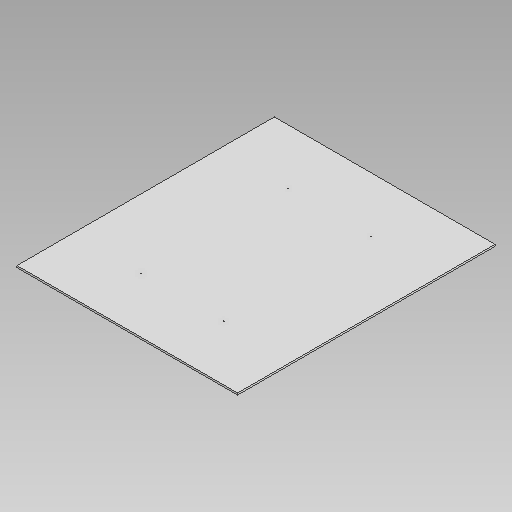
# Autodesk Inventor part: cover_base
Saved by Autodesk Inventor 2021 (Build 250183000, 183)
## iProperties
Created: 2021-05-06
Part Number: cover_base
Material: Generic
Document SubType Name: Modeling
Designer: Watchdog
Density: 1 g/cm^3
Appearance: Default
Author: Watchdog
Autodesk Inventor part; units mm, degrees
ref_plane "YZ Plane" through (0, 0, 0) normal (1, 0, 0) x (0, 1, 0)
ref_plane "XZ Plane" through (0, 0, 0) normal (0, 1, 0) x (-1, 0, 0)
ref_plane "XY Plane" through (0, 0, 0) normal (0, 0, 1) x (1, 0, 0)
sketch "Sketch1" plane through (0, 0, 0) normal (0, 1, 0) x (-1, 0, 0)
  line L0 (600, 700) -> (-600, 700)
  line L1 (-600, 700) -> (-600, -700)
  line L2 (-600, -700) -> (600, -700)
  line L3 (600, -700) -> (600, 700)
  point P0 (0, 0)
  dimension "d0" = 700
  dimension "d1" = 1400
  dimension "d2" = 1200
  dimension "d3" = 600
  constraints: 8 end point, 2 parallel, 1 horizontal, 1 perpendicular
  measures "d0" distance from line of point (0, 0) L0
  measures "d1" distance between parallel lines of L2 L0
  measures "d2" distance between parallel lines of L1 L3
  measures "d3" distance from line of point (0, 0) L3
extrude "base" add sketch "Sketch1" along normal blind 10
sketch "Sketch2" plane through (0, 10, 0) normal (0, 1, 0) x (1, 0, 0)
  point P0 (0, 0)
  point P1 (-225, -400)
  point P2 (225, -400)
  point P3 (-225, 400)
  point P4 (225, 400)
  dimension "d10" = 800
  dimension "d11" = 800
  dimension "d12" = 450
  dimension "d13" = 450
  dimension "d14" = 225
  dimension "d15" = 225
  dimension "d16" = 400
  dimension "d17" = 400
  measures "d10" distance of point (-225, 400) point (-225, -400)
  measures "d11" distance of point (225, 400) point (225, -400)
  measures "d12" distance of point (225, -400) point (-225, -400)
  measures "d13" distance of point (225, 400) point (-225, 400)
  measures "d14" horizontal distance of point (0, 0) point (-225, -400)
  measures "d15" horizontal distance of point (0, 0) point (-225, 400)
  measures "d16" vertical distance of point (0, 0) point (-225, -400)
  measures "d17" vertical distance of point (0, 0) point (225, -400)
hole "mountHoles" at (-225, 10, 400) at (225, 10, 400) at (-225, 10, -400) at (225, 10, -400) direction (0, -1, 0) diameter 5 end through all
equation "\"d0\" = 0.5 * d1"
equation "\"d1\" = cover_length_main"
equation "\"d2\" = cover_width_main"
equation "\"d3\" = 0.5 * d2"
equation "\"d4\" = cover_base_thickness"
equation "\"d10\" = cover_mountHole_xSpacing"
equation "\"d11\" = cover_mountHole_xSpacing"
equation "\"d12\" = cover_mountHole_ySpacing"
equation "\"d13\" = cover_mountHole_ySpacing"
equation "\"d14\" = 0.5 * d12"
equation "\"d15\" = 0.5 * d13"
equation "\"d16\" = 0.5 * d10"
equation "\"d17\" = 0.5 * d11"
equation "\"d18\" = cover_mountHole_diameter"
equation "\"rack_tooth_thickness\" = 5"
equation "\"rack_tooth_addendum\" = 5"
equation "\"rack_tooth_dedendum\" = 5"
equation "\"cover_width_main\" = 1200"
equation "\"cover_length_main\" = 1400"
equation "\"cover_base_thickness\" = 10"
equation "\"cover_mountHole_diameter\" = 5"
equation "\"cover_mountHole_xSpacing\" = 800"
equation "\"cover_mountHole_ySpacing\" = 450"
body "Solid1"
